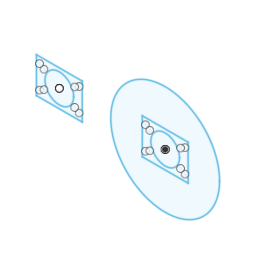
PL servo rotator RS204MD v2 (Autodesk Fusion 360 archive; units mm, degrees)
design "Lighting mount to ZWO filter wheel"
Autodesk Fusion 360 part; units mm, degrees
sketch "スケッチ1" plane through (0, 0, 0) normal (0, 0, 1) x (1, 0, 0)
  circle A0 centre (-34.641, 20) radius 1.5
  circle A1 centre (-34.641, -20) radius 1.5
  circle A2 centre (34.641, 20) radius 1.5
  circle A3 centre (34.641, -20) radius 1.5
  circle A4 centre (0, 0) radius 25
  circle A5 centre (-26.8468, 15.5) radius 1.5
  circle A6 centre (-26.8468, -15.5) radius 1.5
  circle A7 centre (26.8468, 15.5) radius 1.5
  circle A8 centre (26.8468, -15.5) radius 1.5
  line L0 (40, -31) -> (-40, -31)
  line L1 (-40, -31) -> (-40, 31)
  line L2 (-40, 31) -> (40, 31)
  line L3 (40, 31) -> (40, -31)
  circle A9 centre (0, 0) radius 95
  circle A10 centre (-158.0426, -15.5) radius 1.5
  circle A11 centre (-158.0426, 15.5) radius 1.5
  line L4 (-224.8893, 31) -> (-144.8893, 31)
  circle A12 centre (-219.5304, 20) radius 1.5
  circle A13 centre (-219.5304, -20) radius 1.5
  line L5 (-144.8893, 31) -> (-144.8893, -31)
  circle A14 centre (-184.8893, 0) radius 25
  circle A15 centre (-150.2483, 20) radius 1.5
  circle A16 centre (-211.7361, 15.5) radius 1.5
  circle A17 centre (-211.7361, -15.5) radius 1.5
  line L6 (-144.8893, -31) -> (-224.8893, -31)
  circle A18 centre (-150.2483, -20) radius 1.5
  line L7 (-224.8893, -31) -> (-224.8893, 31)
  point P0 (-184.8893, 0)
  point P1 (-184.8893, 0)
  point P2 (-184.8893, 0)
  dimension "d6" = 3
  dimension "d7" = 3
  dimension "d8" = 3
  dimension "d9" = 3
  dimension "d11" = 50
  dimension "d12" = 3
  dimension "d13" = 3
  dimension "d14" = 3
  dimension "d15" = 3
  dimension "d20" = 80
  dimension "d37" = 3
  dimension "d38" = 3
  dimension "d39" = 3
  dimension "d40" = 3
  dimension "d41" = 50
  dimension "d42" = 3
  dimension "d43" = 3
  dimension "d44" = 3
  dimension "d45" = 3
  dimension "d46" = 80
  constraint horizontal L0
  constraint perpendicular L0 L1
  constraint parallel L0 L2
  constraint parallel L1 L3
  constraint horizontal L6
  constraint perpendicular L6 L7
  constraint parallel L4 L6
  constraint parallel L5 L7
  measures "d6" diameter of A0
  measures "d7" diameter of A1
  measures "d8" diameter of A2
  measures "d9" diameter of A3
  measures "d11" diameter of A4
  measures "d12" diameter of A5
  measures "d13" diameter of A6
  measures "d14" diameter of A7
  measures "d15" diameter of A8
  measures "d20" distance of L1.end L2.end
  measures "d37" diameter of A12
  measures "d38" diameter of A13
  measures "d39" diameter of A15
  measures "d40" diameter of A18
  measures "d41" diameter of A14
  measures "d42" diameter of A16
  measures "d43" diameter of A17
  measures "d44" diameter of A11
  measures "d45" diameter of A10
  measures "d46" distance of L4.end L4.start
sketch "スケッチ2" plane through (0, 0, 0) normal (0, 0, 1) x (1, 0, 0)
  line L0 (-6, 73.9298) -> (6, 73.9298)
  line L1 (6, 73.9298) -> (6, 85.9298)
  line L2 (6, 85.9298) -> (-6, 85.9298)
  line L3 (-6, 85.9298) -> (-6, 73.9298)
  circle A0 centre (-7, 79.9298) radius 1.5
  line L4 (0, 83) -> (0, 76)
  circle A1 centre (7, 79.9298) radius 1.5
  circle A2 centre (-18.0423, 78.1808) radius 1.5
  circle A3 centre (-31.357, 73.8546) radius 1.5
  circle A4 centre (-41.3184, 68.779) radius 1.5
  circle A5 centre (-52.6446, 60.55) radius 1.5
  circle A6 centre (-60.55, 52.6446) radius 1.5
  circle A7 centre (-68.779, 41.3184) radius 1.5
  circle A8 centre (-73.8546, 31.357) radius 1.5
  circle A9 centre (-78.1808, 18.0423) radius 1.5
  circle A10 centre (-79.9298, 7) radius 1.5
  circle A11 centre (-79.9298, -7) radius 1.5
  circle A12 centre (-78.1808, -18.0423) radius 1.5
  circle A13 centre (-73.8546, -31.357) radius 1.5
  circle A14 centre (-68.779, -41.3184) radius 1.5
  circle A15 centre (-60.55, -52.6446) radius 1.5
  circle A16 centre (-52.6446, -60.55) radius 1.5
  circle A17 centre (-41.3184, -68.779) radius 1.5
  circle A18 centre (-31.357, -73.8546) radius 1.5
  circle A19 centre (-18.0423, -78.1808) radius 1.5
  circle A20 centre (-7, -79.9298) radius 1.5
  circle A21 centre (7, -79.9298) radius 1.5
  circle A22 centre (18.0423, -78.1808) radius 1.5
  circle A23 centre (31.357, -73.8546) radius 1.5
  circle A24 centre (41.3184, -68.779) radius 1.5
  circle A25 centre (52.6446, -60.55) radius 1.5
  circle A26 centre (60.55, -52.6446) radius 1.5
  circle A27 centre (68.779, -41.3184) radius 1.5
  circle A28 centre (73.8546, -31.357) radius 1.5
  circle A29 centre (78.1808, -18.0423) radius 1.5
  circle A30 centre (79.9298, -7) radius 1.5
  circle A31 centre (79.9298, 7) radius 1.5
  circle A32 centre (78.1808, 18.0423) radius 1.5
  circle A33 centre (73.8546, 31.357) radius 1.5
  circle A34 centre (68.779, 41.3184) radius 1.5
  circle A35 centre (60.55, 52.6446) radius 1.5
  circle A36 centre (52.6446, 60.55) radius 1.5
  circle A37 centre (41.3184, 68.779) radius 1.5
  circle A38 centre (31.357, 73.8546) radius 1.5
  circle A39 centre (18.0423, 78.1808) radius 1.5
  circle A40 centre (-22.2724, 56.076) radius 1.5
  circle A41 centre (-8.7495, 59.6994) radius 1.5
  circle A42 centre (-26.7694, 54.0738) radius 1.5
  circle A43 centre (-38.5108, 46.4488) radius 1.5
  circle A44 centre (-42.1689, 43.155) radius 1.5
  circle A45 centre (-50.9794, 32.275) radius 1.5
  circle A46 centre (-53.4407, 28.012) radius 1.5
  circle A47 centre (-58.4578, 14.9418) radius 1.5
  circle A48 centre (-59.4813, 10.1269) radius 1.5
  circle A49 centre (-60.214, -3.8539) radius 1.5
  circle A50 centre (-59.6994, -8.7495) radius 1.5
  circle A51 centre (-56.076, -22.2724) radius 1.5
  circle A52 centre (-54.0738, -26.7694) radius 1.5
  circle A53 centre (-46.4488, -38.5108) radius 1.5
  circle A54 centre (-43.155, -42.1689) radius 1.5
  circle A55 centre (-32.275, -50.9794) radius 1.5
  circle A56 centre (-28.012, -53.4407) radius 1.5
  circle A57 centre (-14.9418, -58.4578) radius 1.5
  circle A58 centre (-10.1269, -59.4813) radius 1.5
  circle A59 centre (3.8539, -60.214) radius 1.5
  circle A60 centre (8.7495, -59.6994) radius 1.5
  circle A61 centre (22.2724, -56.076) radius 1.5
  circle A62 centre (26.7694, -54.0738) radius 1.5
  circle A63 centre (38.5108, -46.4488) radius 1.5
  circle A64 centre (42.1689, -43.155) radius 1.5
  circle A65 centre (50.9794, -32.275) radius 1.5
  circle A66 centre (53.4407, -28.012) radius 1.5
  circle A67 centre (58.4578, -14.9418) radius 1.5
  circle A68 centre (59.4813, -10.1269) radius 1.5
  circle A69 centre (60.214, 3.8539) radius 1.5
  circle A70 centre (59.6994, 8.7495) radius 1.5
  circle A71 centre (56.076, 22.2724) radius 1.5
  circle A72 centre (54.0738, 26.7694) radius 1.5
  circle A73 centre (46.4488, 38.5108) radius 1.5
  circle A74 centre (43.155, 42.1689) radius 1.5
  circle A75 centre (32.275, 50.9794) radius 1.5
  circle A76 centre (28.012, 53.4407) radius 1.5
  circle A77 centre (14.9418, 58.4578) radius 1.5
  circle A78 centre (10.1269, 59.4813) radius 1.5
  circle A79 centre (-3.8539, 60.214) radius 1.5
  point P0 (0, 79.9298)
  dimension "d47" = 12
  dimension "d48" = 12
  dimension "d49" = 3
  dimension "d52" = 360
  dimension "d61" = 360
  constraint horizontal L0
  constraint perpendicular L0 L1
  constraint parallel L0 L2
  constraint parallel L1 L3
  constraint perpendicular L2 L4
  constraint symmetric A0 L4 A1
  measures "d47" distance of L1.end L2.end
  measures "d48" distance of L0.end L1.end
  measures "d49" diameter of A0
extrude "押し出し5" add sketch "スケッチ1" along normal blind 1 contours L0 L1 L2 L3 | A9 makes body 1
extrude "押し出し6" cut sketch "スケッチ2" along normal blind 10 contours L3 A0 | L3 A0 | L1 A1 | L1 A1 | A2 | A3 | A4 | A5 | A6 | A7 | A8 | A9 | A10 | A11 | A12 | A13 | A14 | A15 | A16 | A17 | A18 | A19 | A20 | A21 | A22 | A23 | A24 | A25 | A26 | A27 | A28 | A29 | A30 | A31 | A32 | A33 | A34 | A35 | A36 | A37 | A38 | A39 bodies 1
extrude "押し出し7" cut sketch "スケッチ2" along normal blind 10 contours A40 | A41 | A42 | A43 | A44 | A45 | A46 | A47 | A48 | A50 | A51 | A52 | A53 | A54 | A55 | A56 | A57 | A58 | A59 | A60 | A61 | A62 | A63 | A64 | A65 | A66 | A67 | A68 | A69 | A70 | A71 | A72 | A73 | A74 | A75 | A76 | A77 | A78 | A79 bodies 1
extrude "押し出し8" add sketch "スケッチ1" along normal blind 5 separate body contours L4 L5 L6 L7 makes body 2
fillet "フィレット1" radius 15 4 edges at (-144.8893, 31, 2.5) (-224.8893, 31, 2.5) (-224.8893, -31, 2.5) (-144.8893, -31, 2.5) on bodies 2
sketch "スケッチ3" plane through (0, 0, 0) normal (0, 0, -1) x (-1, 0, 0)
  circle A0 centre (43.155, -42.1689) radius 1.5
  circle A1 centre (56.076, -22.2724) radius 1.5
  circle A2 centre (50.9794, 32.275) radius 1.5
  circle A3 centre (-26.7694, -54.0738) radius 1.5
  circle A4 centre (-8.7495, -59.6994) radius 1.5
  circle A5 centre (-60.214, 3.8539) radius 1.5
  circle A6 centre (-53.4407, -28.012) radius 1.5
  circle A7 centre (-43.155, 42.1689) radius 1.5
  circle A8 centre (26.7694, 54.0738) radius 1.5
  circle A9 centre (8.7495, 59.6994) radius 1.5
  circle A10 centre (-14.9418, 58.4578) radius 1.5
  circle A11 centre (-28.012, 53.4407) radius 1.5
  circle A12 centre (-56.076, 22.2724) radius 1.5
  circle A13 centre (-50.9794, -32.275) radius 1.5
  circle A14 centre (-3.8539, -60.214) radius 1.5
  circle A15 centre (14.9418, -58.4578) radius 1.5
  circle A16 centre (-42.1689, -43.155) radius 1.5
  circle A17 centre (54.0738, -26.7694) radius 1.5
  circle A18 centre (46.4488, -38.5108) radius 1.5
  circle A19 centre (38.5108, 46.4488) radius 1.5
  circle A20 centre (58.4578, 14.9418) radius 1.5
  circle A21 centre (59.6994, -8.7495) radius 1.5
  circle A22 centre (10.1269, -59.4813) radius 1.5
  circle A23 centre (28.012, -53.4407) radius 1.5
  circle A24 centre (-59.6994, 8.7495) radius 1.5
  circle A25 centre (-58.4578, -14.9418) radius 1.5
  circle A26 centre (-46.4488, 38.5108) radius 1.5
  circle A27 centre (3.8539, 60.214) radius 1.5
  circle A28 centre (22.2724, 56.076) radius 1.5
  circle A29 centre (-10.1269, 59.4813) radius 1.5
  circle A30 centre (-32.275, 50.9794) radius 1.5
  circle A31 centre (-54.0738, 26.7694) radius 1.5
  circle A32 centre (-59.4813, -10.1269) radius 1.5
  circle A33 centre (32.275, -50.9794) radius 1.5
  circle A34 centre (-22.2724, -56.076) radius 1.5
  circle A35 centre (-38.5108, -46.4488) radius 1.5
  circle A36 centre (53.4407, 28.012) radius 1.5
  circle A37 centre (59.4813, 10.1269) radius 1.5
  circle A38 centre (42.1689, 43.155) radius 1.5
  circle A39 centre (-31.357, -73.8546) radius 1.5
  circle A40 centre (73.8546, -31.357) radius 1.5
  circle A41 centre (52.6446, -60.55) radius 1.5
  circle A42 centre (-73.8546, 31.357) radius 1.5
  circle A43 centre (-78.1808, 18.0423) radius 1.5
  circle A44 centre (-78.1808, -18.0423) radius 1.5
  circle A45 centre (78.1808, -18.0423) radius 1.5
  circle A46 centre (31.357, 73.8546) radius 1.5
  circle A47 centre (7, 79.9298) radius 1.5
  circle A48 centre (-60.55, 52.6446) radius 1.5
  circle A49 centre (-7, 79.9298) radius 1.5
  circle A50 centre (60.55, 52.6446) radius 1.5
  circle A51 centre (-41.3184, 68.779) radius 1.5
  circle A52 centre (79.9298, -7) radius 1.5
  circle A53 centre (31.357, -73.8546) radius 1.5
  circle A54 centre (60.55, -52.6446) radius 1.5
  circle A55 centre (68.779, -41.3184) radius 1.5
  circle A56 centre (-73.8546, -31.357) radius 1.5
  circle A57 centre (-79.9298, 7) radius 1.5
  circle A58 centre (-68.779, 41.3184) radius 1.5
  circle A59 centre (-18.0423, -78.1808) radius 1.5
  circle A60 centre (68.779, 41.3184) radius 1.5
  circle A61 centre (41.3184, -68.779) radius 1.5
  circle A62 centre (73.8546, 31.357) radius 1.5
  circle A63 centre (-52.6446, -60.55) radius 1.5
  circle A64 centre (-79.9298, -7) radius 1.5
  circle A65 centre (79.9298, 7) radius 1.5
  circle A66 centre (-31.357, 73.8546) radius 1.5
  circle A67 centre (52.6446, 60.55) radius 1.5
  circle A68 centre (41.3184, 68.779) radius 1.5
  circle A69 centre (-52.6446, 60.55) radius 1.5
  circle A70 centre (18.0423, 78.1808) radius 1.5
  circle A71 centre (-18.0423, 78.1808) radius 1.5
  circle A72 centre (78.1808, 18.0423) radius 1.5
  circle A73 centre (-68.779, -41.3184) radius 1.5
  circle A74 centre (-7, -79.9298) radius 1.5
  circle A75 centre (-60.55, -52.6446) radius 1.5
  circle A76 centre (-41.3184, -68.779) radius 1.5
  circle A77 centre (18.0423, -78.1808) radius 1.5
  circle A78 centre (7, -79.9298) radius 1.5
  circle A79 centre (-26.8468, -15.5) radius 1.5
  circle A80 centre (26.8468, 15.5) radius 1.5
  circle A81 centre (-34.641, 20) radius 1.5
  circle A82 centre (26.8468, -15.5) radius 1.5
  circle A83 centre (-26.8468, 15.5) radius 1.5
  circle A84 centre (34.641, 20) radius 1.5
  circle A85 centre (0, 0) radius 25
  circle A86 centre (34.641, -20) radius 1.5
  circle A87 centre (-34.641, -20) radius 1.5
  circle A88 centre (0, 0) radius 95
  line L0 (1, 33) -> (-1, 33)
  line L1 (-1, 33) -> (-1, 126.8595)
  line L2 (-1, 126.8595) -> (1, 126.8595)
  line L3 (1, 126.8595) -> (1, 33)
  line L4 (1, 33) -> (-1, 126.8595) construction
  line L5 (-1, 33) -> (1, 126.8595) construction
  line L6 (-126.8595, 1) -> (-33, 1)
  line L7 (-33, 1) -> (-33, -1)
  line L8 (-126.8595, -1) -> (-126.8595, 1)
  line L9 (-33, 1) -> (-126.8595, -1) construction
  line L10 (-33, -1) -> (-126.8595, 1) construction
  line L11 (-33, -1) -> (-126.8595, -1)
  line L12 (-1, -126.8595) -> (-1, -33)
  line L13 (-1, -33) -> (1, -33)
  line L14 (1, -126.8595) -> (-1, -126.8595)
  line L15 (-1, -33) -> (1, -126.8595) construction
  line L16 (1, -33) -> (-1, -126.8595) construction
  line L17 (1, -33) -> (1, -126.8595)
  line L18 (126.8595, -1) -> (33, -1)
  line L19 (33, -1) -> (33, 1)
  line L20 (126.8595, 1) -> (126.8595, -1)
  line L21 (33, -1) -> (126.8595, 1) construction
  line L22 (33, 1) -> (126.8595, -1) construction
  line L23 (33, 1) -> (126.8595, 1)
  circle A89 centre (0, 0) radius 49.5177
  circle A90 centre (0, 0) radius 51.5177
  line L24 (96.8736, 82.7315) -> (82.7315, 96.8736)
  line L25 (82.7315, 96.8736) -> (-96.8736, -82.7315)
  line L26 (-96.8736, -82.7315) -> (-82.7315, -96.8736)
  line L27 (-82.7315, -96.8736) -> (96.8736, 82.7315)
  line L28 (96.8736, 82.7315) -> (-96.8736, -82.7315) construction
  line L29 (82.7315, 96.8736) -> (-82.7315, -96.8736) construction
  line L30 (98.2878, -84.1457) -> (84.1457, -98.2878)
  line L31 (84.1457, -98.2878) -> (-98.2878, 84.1457)
  line L32 (-98.2878, 84.1457) -> (-84.1457, 98.2878)
  line L33 (-84.1457, 98.2878) -> (98.2878, -84.1457)
  line L34 (98.2878, -84.1457) -> (-98.2878, 84.1457) construction
  line L35 (84.1457, -98.2878) -> (-84.1457, 98.2878) construction
  point P0 (0, 79.9298)
  point P1 (0, 79.9298)
  point P2 (-79.9298, 0)
  point P3 (-79.9298, 0)
  point P4 (0, -79.9298)
  point P5 (0, -79.9298)
  point P6 (79.9298, 0)
  point P7 (79.9298, 0)
  dimension "d68" = 2
  dimension "d74" = 20
  dimension "d75" = 20
  constraint horizontal L0
  constraint perpendicular L0 L1
  constraint parallel L0 L2
  constraint parallel L1 L3
  constraint coincident L4 P1
  constraint coincident L5 P1
  constraint coincident P1 P0
  constraint perpendicular L24 L25
  constraint parallel L24 L26
  constraint parallel L25 L27
  constraint coincident L28 A85.centre
  constraint coincident L29 A85.centre
  constraint coincident A85.centre A88.centre
  constraint perpendicular L30 L31
  constraint parallel L30 L32
  constraint parallel L31 L33
  constraint coincident L34 A85.centre
  constraint coincident L35 A85.centre
  measures "d68" distance of L1.end L2.end
  measures "d74" distance of L25.end L26.end
  measures "d75" distance of L31.end L32.end
extrude "押し出し10" cut sketch "スケッチ3" against normal blind 5 contours L6 A89 A90 L31 | L1 A89 A90 L33 | L6 L11 A89 A90 | L1 L3 A89 A90 | A88 L6 L11 A90 | L11 A89 A90 L25 | A88 L1 L3 A90 | L3 A89 A90 L25 | L12 A89 A90 L27 | L23 A89 A90 L27 | L17 A89 A90 L31 | L12 L17 A89 A90 | L18 L23 A89 A90 | L18 A89 A90 L33 | A88 L12 L17 A90 | A88 L18 L23 A90 bodies 1
sketch "スケッチ4" plane through (0, 0, 0) normal (0, 0, -1) x (-1, 0, 0)
  circle A0 centre (150.2483, -20) radius 1.5
  circle A1 centre (211.7361, 15.5) radius 1.5
  circle A2 centre (211.7361, -15.5) radius 1.5
  circle A3 centre (158.0426, -15.5) radius 1.5
  circle A4 centre (158.0426, 15.5) radius 1.5
  circle A5 centre (219.5304, -20) radius 1.5
  circle A6 centre (219.5304, 20) radius 1.5
  circle A7 centre (150.2483, 20) radius 1.5
  circle A8 centre (184.8893, 0) radius 25
  arc A9 (144.8893, -16) -> (159.8893, -31) centre (159.8893, -16) ccw
  line L0 (159.8893, -31) -> (209.8893, -31)
  arc A10 (209.8893, -31) -> (224.8893, -16) centre (209.8893, -16) ccw
  line L1 (224.8893, -16) -> (224.8893, 16)
  arc A11 (224.8893, 16) -> (209.8893, 31) centre (209.8893, 16) ccw
  line L2 (209.8893, 31) -> (159.8893, 31)
  arc A12 (159.8893, 31) -> (144.8893, 16) centre (159.8893, 16) ccw
  line L3 (144.8893, 16) -> (144.8893, -16)
  circle A13 centre (184.8893, 0) radius 21
  circle A14 centre (184.8893, 0) radius 18.5
  dimension "d78" = 42
  dimension "d79" = 37
  constraint concentric A8 A13
  constraint concentric A13 A14
  measures "d78" diameter of A13
  measures "d79" diameter of A14
extrude "押し出し11" add sketch "スケッチ4" against normal blind 5 contours A8 | A13 bodies 2
extrude "押し出し12" add sketch "スケッチ4" along normal blind 3 contours A13 bodies 2
sketch "スケッチ5" plane through (0, 0, 0) normal (0, 0, -1) x (-1, 0, 0)
  circle A0 centre (150.2483, 20) radius 3
  circle A1 centre (158.0426, 15.5) radius 3
  circle A2 centre (219.5304, 20) radius 3
  circle A3 centre (211.7361, 15.5) radius 3
  circle A4 centre (158.0426, -15.5) radius 3
  circle A5 centre (150.2483, -20) radius 3
  circle A6 centre (211.7361, -15.5) radius 3
  circle A7 centre (219.5304, -20) radius 3
  point P0 (150.2483, 20)
  point P1 (158.0426, 15.5)
  point P2 (219.5304, 20)
  point P3 (211.7361, 15.5)
  point P4 (158.0426, -15.5)
  point P5 (150.2483, -20)
  point P6 (211.7361, -15.5)
  point P7 (219.5304, -20)
  dimension "d84" = 6
  dimension "d85" = 6
  dimension "d86" = 6
  dimension "d87" = 6
  dimension "d88" = 6
  dimension "d89" = 6
  dimension "d90" = 6
  dimension "d91" = 6
  constraint coincident P0 A0.centre
  constraint coincident P1 A1.centre
  constraint coincident P2 A2.centre
  constraint coincident P3 A3.centre
  constraint coincident P4 A4.centre
  constraint coincident P5 A5.centre
  constraint coincident P6 A6.centre
  constraint coincident P7 A7.centre
  measures "d84" diameter of A0
  measures "d85" diameter of A1
  measures "d86" diameter of A2
  measures "d87" diameter of A3
  measures "d88" diameter of A4
  measures "d89" diameter of A5
  measures "d90" diameter of A6
  measures "d91" diameter of A7
extrude "押し出し13" cut sketch "スケッチ5" against normal blind 3 contours A1 | A2 | A3 bodies 2
extrude "押し出し14" cut sketch "スケッチ5" against normal blind 3 contours A0 | A4 | A5 | A6 | A7 bodies 2
thread "ねじ2" "Camera Filter Metric profile 42.0 M42x0.75 6g" major diameter 41.838 minor diameter 40.912 pitch 0.75 angle 60 modelled right hand crest width 0.1071 on face at (-205.8632, -1.0468, -2) crest through (-205.8083, 0, 0.1875) on bodies 2
extrude "押し出し2" [suppressed]
extrude "押し出し3" [suppressed]
extrude "押し出し4" [suppressed]
hole "穴1" [suppressed]
thread "ねじ1" [suppressed]
